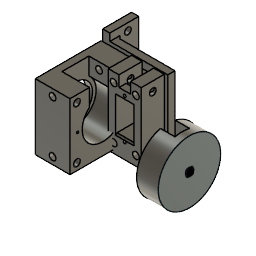
CoupDePouce (Autodesk Fusion 360 design; units mm, degrees)
Autodesk Fusion 360 part; units mm, degrees
note: some values were not read from the file. Chosen so that the rebuilt part matches the saved one: which sketch regions a step uses; where a step ends.
sketch "Esquisse1" plane through (0, 0, 0) normal (0, 1, 0) x (1, 0, 0) in component "SupportBYJ48"
  line L0 (0, 45.5) -> (-45.5, 45.5)
  line L1 (-45.5, 0) -> (0, 0)
  line L2 (0, 0) -> (0, 45.5)
  line L3 (-45.5, 13.45) -> (-33.6128, 13.45)
  line L4 (-33.6128, 32.05) -> (-45.5, 32.05)
  line L5 (-22.75, 22.75) -> (0, 22.75) construction
  arc A0 (-33.6128, 13.45) -> (-33.6128, 32.05) centre (-22.75, 22.75) ccw
  line L6 (-45.5, 45.5) -> (-45.5, 32.05)
  line L7 (-45.5, 13.45) -> (-45.5, 0)
  line L8 (-22.75, 45.5) -> (-22.75, 0) construction
  dimension "d74" = 28.6
  dimension "d81" = 18.6
  dimension "d110" = 45.5
  constraint horizontal L0
  constraint vertical L6
  constraint horizontal L1
  constraint vertical L2
  constraint horizontal L3
  constraint horizontal L4
  constraint coincident L3.start L6
  constraint coincident L1.end L2.start
  constraint coincident L5.start A0.centre
  constraint midpoint L2 L5.end
  constraint symmetric L3.start L4.end L5
  constraint equal L0 L2
  constraint midpoint L0 L8.start
  constraint midpoint L1 L8.end
  constraint coincident L5.start L8
  constraint collinear L6 L7
  measures "d74" diameter of A0
  measures "d81" distance of L3 L4
  measures "d110" distance of L0.start L1.end
extrude "Extrusion1" add sketch "Esquisse1" along normal blind 19 makes body 1 in component "SupportBYJ48"
sketch "Esquisse2" plane through (0, 0, 0) normal (0, -1, 0) x (1, 0, 0) in component "SupportBYJ48"
  line L0 (-45.5, -13.45) -> (-33.6128, -13.45)
  arc A0 (-33.6128, -32.05) -> (-33.6128, -13.45) centre (-22.75, -22.75) ccw
  line L1 (-33.6128, -32.05) -> (-45.5, -32.05)
  line L2 (-45.5, -32.05) -> (-45.5, -45.5)
  line L3 (-45.5, -45.5) -> (0, -45.5)
  line L4 (0, -45.5) -> (0, 0)
  line L5 (0, 0) -> (-45.5, 0)
  line L6 (-45.5, 0) -> (-45.5, -13.45)
  arc A1 (-33.6128, -32.05) -> (-33.6128, -13.45) centre (-22.75, -22.75) ccw
  line L7 (-45.5, 0) -> (0, 0)
  line L8 (0, 0) -> (0, -45.5)
  line L9 (0, 0) -> (-45.5, 0)
  line L10 (-45.5, -45.5) -> (0, -45.5)
  line L11 (0, -45.5) -> (0, 0)
  circle A2 centre (-22.75, -22.75) radius 14.3 construction
  circle A3 centre (-22.75, -22.75) radius 11.8
  line L12 (-45.5, 0) -> (-45.5, -45.5)
  line L13 (-45.5, -13.45) -> (-45.5, 0)
  line L14 (-45.5, -13.45) -> (-45.5, 0)
  constraint horizontal L9
  constraint horizontal L10
  constraint vertical L11
  constraint coincident L4.end L5.start
  constraint concentric A1 A2
  constraint coincident A0.start A2
  constraint coincident L3.end L4.start
  constraint vertical L12
  constraint collinear L12 L14
extrude "Extrusion2" add sketch "Esquisse2" along normal blind 5 bodies 1 in component "SupportBYJ48"
sketch "Esquisse5" plane through (0, 0, 0) normal (0, 0, 1) x (-1, 0, 0) in component "SupportBYJ48"
  line L0 (0, 5) -> (0, -19)
  line L1 (0, -19) -> (45.5, -19)
  line L2 (45.5, -19) -> (45.5, 5)
  line L3 (45.5, 5) -> (0, 5)
  circle A0 centre (4.8, -7) radius 2.3
  circle A1 centre (40.7, -7) radius 2.3
  line L4 (43, -3.3112) -> (43, -15.0162) construction
  line L5 (45.5, 5) -> (45.5, -19)
  line L6 (0, 5) -> (0, -19)
  line L7 (45.5, -7) -> (0, -7) construction
  line L8 (2.5, -3) -> (2.5, -12) construction
  dimension "d112" = 2.5
  dimension "d113" = 4.6
  dimension "d114" = 2.5
  dimension "espace_trou_patte" = 35.9
  constraint tangent A1 L4
  constraint vertical L4
  constraint equal A0 A1
  constraint midpoint L5 L7.start
  constraint midpoint L6 L7.end
  constraint coincident A1.centre L7
  constraint coincident A0.centre L7
  constraint tangent A0 L8
  constraint vertical L8
  measures "d112" distance of L4 L5
  measures "d113" diameter of A1
  measures "d114" distance of L6 L8
  measures "espace_trou_patte" distance of A0.centre A1.centre
extrude "Extrusion5" cut sketch "Esquisse5" against normal up to surface (45.5 mm away) contours A0 | A1 bodies 1 in component "SupportBYJ48"
sketch "Esquisse6" plane through (0, 19, 0) normal (0, 1, 0) x (-1, 0, 0) in component "SupportBYJ48"
  line L0 (33.6128, -13.45) -> (45.5, -13.45)
  line L1 (45.5, -13.45) -> (45.5, 0)
  line L2 (45.5, 0) -> (0, 0)
  line L3 (0, 0) -> (0, -45.5)
  line L4 (0, -45.5) -> (45.5, -45.5)
  line L5 (45.5, -45.5) -> (45.5, -32.05)
  line L6 (45.5, -32.05) -> (33.6128, -32.05)
  arc A0 (33.6128, -13.45) -> (33.6128, -32.05) centre (22.75, -22.75) ccw
  circle A1 centre (40.7, -40.7) radius 2.3
  circle A2 centre (4.8, -40.7) radius 2.3
  circle A3 centre (40.7, -4.8) radius 2.3
  circle A4 centre (4.8, -4.8) radius 2.3
  line L7 (45.5, -45.5) -> (45.5, -32.05)
  line L8 (0, -45.5) -> (45.5, -45.5)
  line L9 (0, 0) -> (0, -45.5)
  line L10 (45.5, 0) -> (0, 0)
  line L11 (45.5, -13.45) -> (45.5, 0)
  line L12 (43, -43) -> (43, -37.0409) construction
  line L13 (43, -43) -> (37.7131, -43) construction
  line L14 (0, -22.75) -> (45, -22.75) construction
  line L15 (22.75, -45.5) -> (22.75, 0) construction
  dimension "d118" = 4.6
  dimension "d120" = 2.5
  dimension "d121" = 2.5
  constraint equal A1 A3
  constraint equal A3 A4
  constraint equal A2 A4
  constraint vertical L12
  constraint perpendicular L12 L13
  constraint tangent A1 L13
  constraint tangent A1 L12
  constraint midpoint L9 L14.start
  constraint perpendicular L9 L14
  constraint midpoint L8 L15.start
  constraint midpoint L10 L15.end
  constraint symmetric A1.centre A2.centre L15
  constraint symmetric A2.centre A4.centre L14
  constraint symmetric A1.centre A3.centre L14
  measures "d118" diameter of A1
  measures "d120" distance of L7 L12
  measures "d121" distance of L8 L13
extrude "Extrusion6" cut sketch "Esquisse6" against normal up to surface (24 mm away) contours A1 | A2 | A3 | A4 bodies 1 in component "SupportBYJ48"
sketch "Esquisse7" plane through (0, 19, 0) normal (0, 1, 0) x (-1, 0, 0) in component "SupportBYJ48"
  circle A0 centre (4.8, -40.7) radius 2.3
  circle A1 centre (40.7, -4.8) radius 2.3
  circle A2 centre (40.7, -40.7) radius 2.3
  circle A3 centre (4.8, -4.8) radius 2.3
  line L0 (33.6128, -13.45) -> (45.5, -13.45)
  line L1 (45.5, -13.45) -> (45.5, 0)
  line L2 (45.5, 0) -> (0, 0)
  line L3 (0, 0) -> (0, -45.5)
  line L4 (0, -45.5) -> (45.5, -45.5)
  line L5 (45.5, -45.5) -> (45.5, -32.05)
  line L6 (45.5, -32.05) -> (33.6128, -32.05)
  arc A4 (33.6128, -13.45) -> (33.6128, -32.05) centre (22.75, -22.75) ccw
  circle A5 centre (22.75, -40.25) radius 0.75
  circle A6 centre (22.75, -5.25) radius 0.75
  arc A7 (33.6128, -13.45) -> (33.6128, -32.05) centre (22.75, -22.75) ccw
  line L7 (22.75, -22.75) -> (8.45, -22.75) construction
  dimension "d124" = 35
  dimension "d125" = 1.5
  constraint equal A5 A6
  constraint vertical A5.centre A6.centre
  constraint vertical A4.centre A5.centre
  constraint coincident A4.centre A7.centre
  constraint midpoint A4 L7.end
  constraint symmetric A5.centre A6.centre L7
  measures "d124" vertical distance of A5.centre A6.centre
  measures "d125" diameter of A5
extrude "Extrusion7" cut sketch "Esquisse7" against normal up to surface (19 mm away) contours A5 | A6 bodies 1 in component "SupportBYJ48"
sketch "Esquisse1 (2)" plane through (0, 0, 0) normal (0, 1, 0) x (1, 0, 0) in component "SupportFT90B_boite"
  line L0 (0, 0) -> (0, -48.9)
  line L1 (0, -48.9) -> (7.35, -48.9)
  line L2 (7.35, -48.9) -> (7.35, -36.3)
  line L3 (7.35, -36.3) -> (5, -36.3)
  line L4 (5, -36.3) -> (5, -12.6)
  line L5 (5, -12.6) -> (17.7, -12.6)
  line L6 (17.7, -12.6) -> (17.7, -36.3)
  line L7 (17.7, -36.3) -> (15.35, -36.3)
  line L8 (15.35, -36.3) -> (15.35, -48.9)
  line L9 (15.35, -48.9) -> (22.7, -48.9)
  line L10 (22.7, -48.9) -> (22.7, 0)
  line L11 (22.7, 0) -> (0, 0)
  line L12 (11.35, -12.6) -> (11.35, 0) construction
  line L13 (22.7, -24.45) -> (0, -24.45) construction
  dimension "d14" = 23.7
  dimension "d15" = 12.7
  dimension "d16" = 5
  dimension "d17" = 8
  dimension "d70" = 5
  dimension "d131" = 48.9
  constraint vertical L0
  constraint perpendicular L0 L1
  constraint perpendicular L1 L2
  constraint perpendicular L2 L3
  constraint perpendicular L3 L4
  constraint perpendicular L4 L5
  constraint perpendicular L5 L6
  constraint perpendicular L4 L7
  constraint perpendicular L7 L8
  constraint perpendicular L4 L9
  constraint perpendicular L9 L10
  constraint perpendicular L0 L11
  constraint coincident L0.start L11.end
  constraint collinear L1 L9
  constraint collinear L3 L7
  constraint midpoint L5 L12.start
  constraint coincident L11 L12.end
  constraint perpendicular L11 L12
  constraint symmetric L2.end L7.end L12
  constraint midpoint L10 L13.start
  constraint midpoint L0 L13.end
  constraint symmetric L5.end L6.end L13
  measures "d14" distance of L5.end L6.end
  measures "d15" distance of L4.end L5.end
  measures "d16" distance of L0 L4
  measures "d17" distance of L2 L8
  measures "d70" distance of L6 L10
  measures "d131" distance of L0.start L0.end
extrude "Extrusion1'" add sketch "Esquisse1 (2)" along normal blind 16 separate body makes body 2 in component "SupportFT90B_boite"
sketch "Esquisse3" plane through (0, 0, 0) normal (-1, 0, 0) x (0, -1, 0) in component "SupportFT90B_boite"
  line L0 (-16, 0) -> (0, 0)
  line L1 (0, 0) -> (0, 48.9)
  line L2 (0, 48.9) -> (-16, 48.9)
  line L3 (0, 48.9) -> (-16, 48.9)
  line L4 (0, 48.9) -> (0, 36.3)
  line L5 (0, 36.3) -> (-5, 36.3)
  line L6 (-5, 36.3) -> (-5, 41.3)
  line L7 (-5, 41.3) -> (0, 41.3)
  line L8 (0, 41.3) -> (0, 36.3)
  line L9 (-16, 48.9) -> (-16, 0)
  dimension "d26" = 5
  constraint horizontal L5
  constraint vertical L6
  constraint horizontal L7
  constraint vertical L8
  constraint coincident L4.end L5.start
  constraint equal L7 L8
  measures "d26" distance of L4.end L7.end
extrude "Extrusion3" add sketch "Esquisse3" against normal up to surface (22.7 mm away) contours L1 L4 L5 L6 L7 L8 bodies 2 in component "SupportFT90B_boite"
chamfer "Chanfrein1" distance 2 angle 45 1 edges at (11.35, 5, 36.3) on bodies 2 in component "SupportFT90B_boite"
sketch "Esquisse4" plane through (0, 0, 0) normal (0, -1, 0) x (1, 0, 0) in component "SupportFT90B_boite"
  line L0 (5, 36.3) -> (17.7, 36.3)
  line L1 (17.7, 36.3) -> (17.7, 12.6)
  line L2 (17.7, 12.6) -> (5, 12.6)
  line L3 (5, 12.6) -> (5, 36.3)
  line L4 (22.7, 0) -> (22.7, 48.9)
  line L5 (15.35, 41.3) -> (7.35, 41.3)
  line L6 (0, 0) -> (22.7, 0)
  line L7 (7.35, 41.3) -> (15.35, 41.3)
  line L8 (22.7, 0) -> (0, 0)
  circle A0 centre (11.35, 38.3) radius 0.95
  circle A1 centre (11.35, 10.6) radius 0.95
  line L9 (22.7, 48.9) -> (22.7, 0) construction
  line L10 (0, 0) -> (0, 48.9) construction
  line L11 (17.7, 12.6) -> (17.7, 36.3)
  line L12 (17.7, 36.3) -> (5, 36.3)
  line L13 (17.7, 24.45) -> (5, 24.45) construction
  line L14 (11.35, 36.3) -> (11.35, 12.6) construction
  line L15 (7.35, 41.3) -> (7.35, 48.9)
  line L16 (7.35, 48.9) -> (0, 48.9)
  line L17 (22.7, 48.9) -> (15.35, 48.9)
  line L18 (15.35, 48.9) -> (15.35, 41.3)
  line L19 (0, 48.9) -> (0, 0)
  circle A2 centre (19.025, 6.5) radius 2.3
  line L20 (17.7, 24.45) -> (5, 24.45) construction
  circle A3 centre (19.025, 42.4) radius 2.3
  circle A4 centre (3.675, 6.5) radius 2.3
  circle A5 centre (3.675, 42.4) radius 2.3
  line L21 (19.025, 48.9) -> (19.025, 37) construction
  dimension "d31" = 1.9
  dimension "d34" = 27.7
  dimension "d133" = 4.6
  dimension "d142" = 35.9
  constraint equal A0 A1
  constraint midpoint L11 L13.start
  constraint midpoint L3 L13.end
  constraint midpoint L12 L14.start
  constraint midpoint L2 L14.end
  constraint symmetric A0.centre A1.centre L13
  constraint coincident A0.centre L14
  constraint symmetric L20.start L13 L13.start
  constraint symmetric L20.end L13 L13.end
  constraint equal A2 A4
  constraint equal A2 A3
  constraint equal A2 A5
  constraint horizontal A3.centre A5.centre
  constraint vertical A4.centre A5.centre
  constraint horizontal A2.centre A4.centre
  constraint symmetric L13 A4.centre A5.centre
  constraint vertical A2.centre A3.centre
  constraint symmetric L14 A2.centre A4.centre
  constraint midpoint L17 L21.start
  constraint perpendicular L17 L21
  constraint coincident A3.centre L21
  measures "d31" diameter of A0
  measures "d34" distance of A0.centre A1.centre
  measures "d133" diameter of A2
  measures "d142" distance of A4.centre A5.centre
extrude "Extrusion4" cut sketch "Esquisse4" against normal up to surface (5 mm away) contours A0 | A1 bodies 2 in component "SupportFT90B_boite"
chamfer "Chanfrein2" distance 1 angle 45 1 edges at (11.35, 0, 12.6) on bodies 2 in component "SupportFT90B_boite"
sketch "Esquisse1 (3)" plane through (0, 0, 0) normal (0, 1, 0) x (1, 0, 0) in component "Patte_fixation"
  line L0 (0, 0) -> (-40, 0)
  line L1 (-40, 0) -> (-40, -50.5)
  line L2 (-40, -50.5) -> (0, -50.5)
  line L3 (0, -50.5) -> (0, 0)
  line L4 (-6, -40.9) -> (-34, -40.9)
  arc A0 (-34, -40.9) -> (-34, -45.5) centre (-34, -43.2) ccw
  line L5 (-34, -45.5) -> (-6, -45.5)
  arc A1 (-6, -45.5) -> (-6, -40.9) centre (-6, -43.2) ccw
  line L6 (-6, -43.2) -> (-34, -43.2) construction
  line L7 (-6, -5) -> (-34, -5)
  arc A2 (-34, -5) -> (-34, -9.6) centre (-34, -7.3) ccw
  line L8 (-34, -9.6) -> (-6, -9.6)
  arc A3 (-6, -9.6) -> (-6, -5) centre (-6, -7.3) ccw
  line L9 (-6, -7.3) -> (-34, -7.3) construction
  line L10 (-20, -50.5) -> (-20, 0) construction
  line L11 (-40, -25.25) -> (0, -25.25) construction
  dimension "d44" = 40
  dimension "d45" = 28
  dimension "d46" = 2.3
  dimension "d47" = 35.9
  dimension "d129" = 5
  constraint horizontal L0
  constraint vertical L1
  constraint horizontal L2
  constraint vertical L3
  constraint coincident L0.start L3.end
  constraint tangent L4 A0
  constraint tangent A0 L5
  constraint parallel L4 L5
  constraint tangent L5 A1
  constraint tangent L4 A1
  constraint horizontal L6
  constraint tangent L7 A2
  constraint tangent A2 L8
  constraint parallel L7 L8
  constraint tangent L8 A3
  constraint tangent L7 A3
  constraint horizontal L9
  constraint midpoint L2 L10.start
  constraint midpoint L0 L10.end
  constraint midpoint L1 L11.start
  constraint midpoint L3 L11.end
  constraint symmetric A1.centre A0.centre L10
  constraint symmetric A3.centre A2.centre L10
  constraint equal A0 A2
  constraint equal L6 L9
  constraint symmetric A0.centre A2.centre L11
  measures "d44" distance of L1.end L2.end
  measures "d45" distance of A1.centre A0.centre
  measures "d46" radius of A0
  measures "d47" distance of A0.centre A2.centre
  measures "d129" distance of L0 L7
extrude "Extrusion1''" add sketch "Esquisse1 (3)" along normal blind 5 separate body makes body 3 in component "Patte_fixation"
sketch "Esquisse2 (2)" plane through (0, 0, 0) normal (0, -1, 0) x (1, 0, 0) in component "Patte_fixation"
  arc A0 (-6, 40.9) -> (-6, 45.5) centre (-6, 43.2) ccw
  line L0 (-6, 40.9) -> (-34, 40.9)
  arc A1 (-34, 45.5) -> (-34, 40.9) centre (-34, 43.2) ccw
  line L1 (-34, 45.5) -> (-6, 45.5)
  arc A2 (-6, 5) -> (-6, 9.6) centre (-6, 7.3) ccw
  line L2 (-6, 5) -> (-34, 5)
  arc A3 (-34, 9.6) -> (-34, 5) centre (-34, 7.3) ccw
  line L3 (-34, 9.6) -> (-6, 9.6)
  line L4 (0, 0) -> (0, 50.5)
  line L5 (0, 50.5) -> (-40, 50.5)
  line L6 (-40, 50.5) -> (-40, 0)
  line L7 (-40, 0) -> (0, 0)
  line L8 (-40, 0) -> (-40, 50.5)
  line L9 (-40, 55.5) -> (-45, 55.5)
  line L10 (-45, 55.5) -> (-45, -5)
  line L11 (-45, -5) -> (-40, -5)
  line L12 (-40, -5) -> (-40, 55.5)
  dimension "d50" = 5
  dimension "d55" = 5
  dimension "d130" = 5
  constraint horizontal L9
  constraint vertical L10
  constraint horizontal L11
  constraint vertical L12
  constraint coincident L9.start L12.end
  constraint collinear L8 L12
  measures "d50" distance of L9.start L9.end
  measures "d55" distance of L6.end L11.end
  measures "d130" distance of L5.end L9.start
extrude "Extrusion2'" add sketch "Esquisse2 (2)" against normal blind 20 contours L6 L8 L9 L10 L11 L12 bodies 3 in component "Patte_fixation"
sketch "Esquisse4 (2)" plane through (-40, 0, 0) normal (1, 0, 0) x (0, 1, 0) in component "Patte_fixation"
  line L0 (5, 50.5) -> (5, 0)
  line L1 (5, 0) -> (0, 0)
  line L2 (0, 0) -> (0, -5)
  line L3 (0, -5) -> (20, -5)
  line L4 (20, -5) -> (20, 55.5)
  line L5 (20, 55.5) -> (0, 55.5)
  line L6 (5, 0) -> (5, 50.5)
  line L7 (20, 55.5) -> (20, -5)
  line L8 (5, 0) -> (20, 0) construction
  line L9 (5, 50.5) -> (20, 50.5) construction
  line L10 (12.5, 50.5) -> (12.5, 0) construction
  circle A0 centre (12.5, 0) radius 2.3
  circle A1 centre (12.5, 50.5) radius 2.3
  line L11 (0, 50.5) -> (5, 50.5)
  line L12 (0, 55.5) -> (0, 50.5)
  dimension "d57" = 4.6
  dimension "d58" = 4.6
  constraint coincident L0.end L1.start
  constraint coincident L7 L8.end
  constraint perpendicular L7 L8
  constraint coincident L0.start L6.end
  constraint perpendicular L7 L9
  constraint midpoint L9 L10.start
  constraint midpoint L8 L10.end
  constraint perpendicular L8 L10
  constraint coincident L10.end A0.centre
  constraint coincident L10.start A1.centre
  measures "d57" diameter of A0
  measures "d58" diameter of A1
extrude "Extrusion3'" cut sketch "Esquisse4 (2)" against normal up to surface (5 mm away) contours A0 | A1 bodies 3 in component "Patte_fixation"
chamfer "Chanfrein1'" distance 2 angle 45 1 edges at (-40, 5, 25.25) on bodies 3 in component "Patte_fixation"
ref_plane "Plan de construction1" through (-20, 2.5, 25.25) normal (0, 0, -1) x (-1, 0, 0) in component "Patte_fixation"
sketch "Esquisse5 (2)" plane through (0, 0, 25.25) normal (0, 0, -1) x (-1, 0, 0) in component "Patte_fixation"
  line L0 (0, 5) -> (38, 5)
  line L1 (40, 0) -> (40, 20)
  line L2 (40, 20) -> (0, 5)
  line L3 (0, 5) -> (40, 5)
  line L4 (40, 5) -> (40, 20)
  constraint coincident L1.end L2.start
  constraint coincident L0.start L2.end
  constraint perpendicular L3 L4
  constraint collinear L0 L3
extrude "Extrusion4'" add sketch "Esquisse5 (2)" along normal mid plane 2.5 bodies 3 in component "Patte_fixation"
extrude "Extrusion6'" cut sketch "Esquisse4" against normal up to surface (16 mm away) contours A2 | A3 | A4 | A5 bodies 2 in component "SupportFT90B_boite"
sketch "Esquisse6 (2)" plane through (0, 0, 0) normal (-1, 0, 0) x (0, -1, 0) in component "SupportFT90B_boite"
  line L0 (0, 0) -> (0, 48.9)
  line L1 (0, 48.9) -> (-16, 48.9)
  line L2 (-16, 48.9) -> (-16, 0)
  line L3 (-16, 0) -> (0, 0)
  line L4 (0, 0) -> (0, 48.9)
  line L5 (0, 48.9) -> (-16, 48.9)
  line L6 (0, 24.45) -> (-16, 24.45) construction
  line L7 (-8, 48.9) -> (-8, 0) construction
  circle A0 centre (-8, 6.5) radius 2.3
  circle A1 centre (-8, 42.4) radius 2.3
  dimension "d138" = 4.6
  dimension "d139" = 35.9
  constraint midpoint L4 L6.start
  constraint midpoint L2 L6.end
  constraint midpoint L5 L7.start
  constraint midpoint L3 L7.end
  constraint coincident L7 A0.centre
  constraint coincident L7 A1.centre
  constraint equal A0 A1
  constraint symmetric L6 A0.centre A1.centre
  measures "d138" diameter of A0
  measures "d139" distance of A0.centre A1.centre
extrude "Extrusion7'" cut sketch "Esquisse6 (2)" along normal up to far side of body 2 contours A0 | A1 bodies 2 in component "SupportFT90B_boite"
sketch "Esquisse1 (4)" plane through (0, 0, 0) normal (1, 0, 0) x (0, 1, 0) in component "Bouton_rotatif_BYJ48"
  circle A0 centre (0, 0) radius 21.55
  dimension "d155" = 43.1
  constraint coincident A0.centre origin
  measures "d155" diameter of A0
extrude "Extrusion1'''" add sketch "Esquisse1 (4)" along normal blind 15 separate body makes body 4 in component "Bouton_rotatif_BYJ48"
sketch "Esquisse2 (3)" plane through (0, 0, 0) normal (1, 0, 0) x (0, 1, 0) in component "Bouton_rotatif_BYJ48"
  line L0 (-5, 20.9619) -> (-5, -20.9619)
  line L1 (5, -20.9619) -> (5, 20.9619)
  line L2 (5, 20.9619) -> (-5, -20.9619) construction
  line L3 (-5, 20.9619) -> (5, -20.9619) construction
  circle A0 centre (0, 0) radius 21.55
  arc A1 (-5, -20.9619) -> (5, -20.9619) centre (0, 0) ccw
  arc A2 (5, 20.9619) -> (-5, 20.9619) centre (0, 0) ccw
  dimension "d160" = 10
  constraint parallel L0 L1
  constraint coincident L2 A0.centre
  constraint coincident L3 A0.centre
  constraint coincident A0.centre A1.centre
  constraint coincident L1.end A0
  constraint concentric A1 A2
  measures "d160" distance of L0 L1
extrude "Extrusion2''" cut sketch "Esquisse2 (3)" along normal blind 10 contours L0 L1 A0 A1 A2 bodies 4 in component "Bouton_rotatif_BYJ48"
sketch "Esquisse3 (2)" plane through (15, 0, 0) normal (1, 0, 0) x (0, 1, 0) in component "Bouton_rotatif_BYJ48"
  circle A0 centre (0, 0) radius 21.55
  circle A1 centre (0, 0) radius 2.65
  line L0 (1.65, 2.0736) -> (-1.65, 2.0736)
  line L1 (-1.65, 2.0736) -> (-1.65, -2.0736)
  line L2 (-1.65, -2.0736) -> (1.65, -2.0736)
  line L3 (1.65, -2.0736) -> (1.65, 2.0736)
  line L4 (1.65, 2.0736) -> (-1.65, -2.0736) construction
  line L5 (-1.65, 2.0736) -> (1.65, -2.0736) construction
  dimension "d165" = 5.3
  dimension "d166" = 3.3
  constraint coincident A0.centre A1.centre
  constraint horizontal L0
  constraint perpendicular L0 L1
  constraint parallel L0 L2
  constraint parallel L1 L3
  constraint coincident L4 A0.centre
  constraint coincident L5 A0.centre
  constraint coincident A1 L0.start
  measures "d165" diameter of A1
  measures "d166" distance of L1 L3
extrude "Extrusion3''" cut sketch "Esquisse3 (2)" against normal blind 1 contours A1 L3 | A1 L0 | L0 L1 L2 L3 | A1 L2 | A1 L1 bodies 4 in component "Bouton_rotatif_BYJ48"
extrude "Extrusion4''" cut sketch "Esquisse3 (2)" against normal blind 10 contours A1 L0 | L0 L1 L2 L3 | A1 L2 bodies 4 in component "Bouton_rotatif_BYJ48"
component "SupportBYJ48" placed x (0, 0, -1) y (1, 0, 0) z (0, -1, 0) at (-41, -45.5, 2.5)
component "SupportFT90B_boite" placed x (1, 0, 0) y (0, 1, 0) z (0, 0, 1) at (-25.025, -16, 0.8)
component "Patte_fixation" placed x (1, 0, 0) y (0, 1, 0) z (0, 0, 1) at (0, 0, 0)
component "Patte_fixation" placed x (1, 0, 0) y (0, -1, 0) z (0, 0, -1) at (0, -45.5, 50.5)
component "Bouton_rotatif_BYJ48" placed x (1, 0, 0) y (0, 1, 0) z (0, 0, 1) at (0, 0, 0)
equation "hauteur_FT90B = 22.5 mm"
equation "jeu_3D = 0.3 mm"
equation "epaisseur_plastique = 5 mm"
equation "epaisseur_FT90B = 12.1 mm"
equation "hauteur_patte_fixation = 10 mm"
equation "largeur_FT90B = 15.7 mm"
equation "d14 = hauteur_FT90B + 2 * jeu_3D + jeu_assemblage_FT90B"
equation "d15 = epaisseur_FT90B + 2 * jeu_3D"
equation "d16 = epaisseur_plastique"
equation "d17 = largeur_fil_FT90B"
equation "largeur_fil_FT90B = 8 mm"
equation "d19 = largeur_FT90B + jeu_3D"
equation "epaisseur_plastique_haut = 2 mm"
equation "d26 = epaisseur_plastique"
equation "diam_perçage_FT90B = 2.2 mm"
equation "d31 = diam_perçage_FT90B - jeu_3D"
equation "espace_trous_FT90B = 27.7 mm"
equation "d34 = espace_trous_FT90B"
equation "espace_trous_patte = 30 mm"
equation "diam_vis_patte = 4 mm"
equation "longueur_patte_reglage = 40 mm"
equation "d44 = longueur_patte_reglage"
equation "d45 = longueur_patte_reglage - 3 * diam_vis_patte"
equation "d46 = ( diam_vis_patte + jeu_vis ) / 2"
equation "d47 = espace_trou_patte"
equation "d48 = epaisseur_plastique"
equation "d50 = epaisseur_plastique"
equation "d51 = -longueur_patte_reglage / 2"
equation "d55 = epaisseur_plastique"
equation "d57 = diam_vis_patte + 2 * jeu_3D"
equation "d58 = diam_vis_patte + 2 * jeu_3D"
equation "jeu_assemblage_FT90B = 0.6 mm"
equation "epaisseur_plastique_min = 2.5 mm"
equation "d70 = epaisseur_plastique"
equation "diam_boitier_BYJ48 = 28 mm"
equation "d74 = diam_boitier_BYJ48 + 2 * jeu_3D"
equation "BYJ48_largeur_fil = 18 mm"
equation "d81 = BYJ48_largeur_fil + 2 * jeu_3D"
equation "BYJ48_epaisseur_boitier = 19 mm"
equation "d84 = BYJ48_epaisseur_boitier"
equation "d86 = -epaisseur_plastique_min"
equation "BYJ48_rebord_fond_support = 3 mm"
equation "d88 = epaisseur_plastique"
equation "BYJ48_entre_trous_fixation = 35 mm"
equation "d108 = epaisseur_plastique_min"
equation "d110 = BYJ48_entre_trous_fixation + BYJ48_hauteur_patte * 1.5"
equation "BYJ48_hauteur_patte = 7 mm"
equation "d112 = epaisseur_plastique_min"
equation "d113 = diam_vis_patte + jeu_vis"
equation "d114 = epaisseur_plastique_min"
equation "d118 = diam_vis_patte + jeu_vis"
equation "jeu_vis = 0.6 mm"
equation "d120 = epaisseur_plastique_min"
equation "d121 = epaisseur_plastique_min"
equation "d124 = BYJ48_entre_trous_fixation"
equation "d125 = BYJ48_diam_percage_fixation"
equation "BYJ48_diam_percage_fixation = 1.5 mm"
equation "d129 = epaisseur_plastique"
equation "d130 = epaisseur_plastique"
equation "d131 = espace_trou_patte + 2 * ( diam_vis_patte + epaisseur_plastique_min )"
equation "d133 = jeu_vis + diam_vis_patte"
equation "d138 = diam_vis_patte + jeu_vis"
equation "d139 = espace_trou_patte"
equation "d142 = espace_trou_patte"
equation "d155 = ( BYJ48_entre_trous_fixation + BYJ48_hauteur_patte * 1.5 ) - 4 * jeu_assemblage_FT90B"
equation "largeur_levier_bouton = 10 mm"
equation "d158 = largeur_levier_bouton + epaisseur_plastique"
equation "d160 = largeur_levier_bouton"
equation "d161 = largeur_levier_bouton"
equation "BYJ48_diam_axe = 5 mm"
equation "BYJ48_epaisseur_plat_axe = 3 mm"
equation "d165 = BYJ48_diam_axe + jeu_3D"
equation "d166 = BYJ48_epaisseur_plat_axe + jeu_3D"
named bodies: "Support_FT90B", "Patte_fixation", "Support_BYJ48", "Bouton_rotatif_BYJ48"
